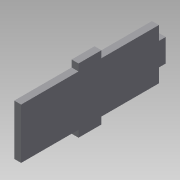
# Autodesk Inventor part: Side
Saved by Autodesk Inventor 2013 (Build 170138000, 138)
## iProperties
Created: 2013-12-12
Part Number: Side
Material: Generic
Document SubType Name: Modeling
Designer: Eric
Density: 1 g/cm^3
Author: Eric
Autodesk Inventor part; units mm, degrees
ref_plane "YZ Plane" through (0, 0, 0) normal (1, 0, 0) x (0, 1, 0)
ref_plane "XZ Plane" through (0, 0, 0) normal (0, 1, 0) x (-1, 0, 0)
ref_plane "XY Plane" through (0, 0, 0) normal (0, 0, 1) x (1, 0, 0)
sketch "Sketch1" plane through (0, 0, 0) normal (1, 0, 0) x (0, 1, 0)
  line L0 (28, 22) -> (28, 25)
  line L1 (28, 25) -> (38, 25)
  line L2 (38, 25) -> (38, 22)
  line L3 (63, 22) -> (38, 22)
  line L4 (28, 22) -> (3, 22)
  line L5 (28, 0) -> (28, -3)
  line L6 (28, -3) -> (38, -3)
  line L7 (38, -3) -> (38, 0)
  line L8 (3, 0) -> (28, 0)
  line L9 (38, 0) -> (63, 0)
  line L10 (66, 16) -> (63, 16)
  line L11 (63, 6) -> (66, 6)
  line L12 (3, 22) -> (3, 0)
  line L13 (63, 16) -> (63, 22)
  line L14 (63, 6) -> (63, 0)
  line L15 (66, 16) -> (66, 6)
  dimension "d2" = 3
  dimension "d3" = 10
  dimension "d5" = 3
  dimension "d6" = 3
  dimension "d11" = 3
  dimension "d12" = 10
  dimension "d19" = 22
  dimension "d23" = 6
  dimension "d24" = 10
  dimension "d25" = 6
  dimension "d26" = 25
  dimension "d27" = 25
  dimension "d28" = 25
  dimension "d29" = 10
  dimension "d30" = 25
  constraints: 32 end point, 10 perpendicular, 5 parallel, 2 horizontal, 1 horizontal alignment
  measures "d2" distance of L0.start L0.end
  measures "d3" distance of L0.end L1.end
  measures "d5" distance of L5.start L5.end
  measures "d6" distance of L6.end L7.end
  measures "d11" distance of L10.start L10.end
  measures "d12" distance of L10.end L11.start
  measures "d19" distance between parallel lines of L8 L4
  measures "d23" distance of L10.end L3.start
  measures "d24" distance of L10.start L11.end
  measures "d25" distance of L11.start L9.end
  measures "d26" distance of L4.end L0.start
  measures "d27" distance of L3.start L2.end
  measures "d28" distance of L7.end L9.end
  measures "d29" distance of L5.end L6.end
  measures "d30" distance of L8.start L5.start
extrude "Extrusion1" add sketch "Sketch1" along normal blind 3
body "Solid1"
